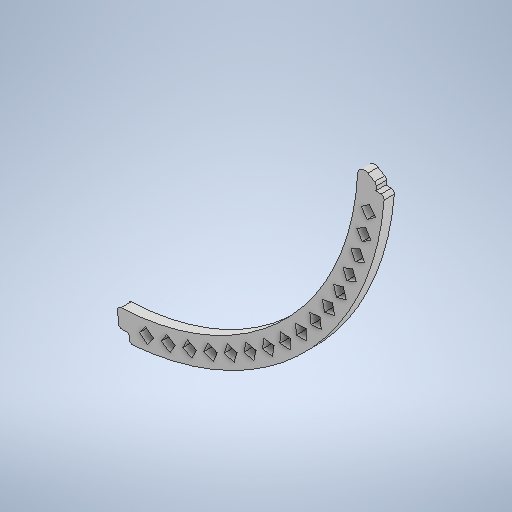
# Autodesk Inventor part: shim_cartridge_V4
Saved by Autodesk Inventor 2025.2 (Build 292293000, 293)
## iProperties
Created: 2024-04-08
Part Number: shim_cartridge_V4
Material: Generic
Document SubType Name: Modeling
Designer: Joshua Harper
Density: 1 g/cm^3
Appearance: Default
Author: Joshua Harper
Autodesk Inventor part; units mm, degrees
ref_plane "YZ Plane" through (0, 0, 0) normal (1, 0, 0) x (0, 1, 0)
ref_plane "XZ Plane" through (0, 0, 0) normal (0, 1, 0) x (-1, 0, 0)
ref_plane "XY Plane" through (0, 0, 0) normal (0, 0, 1) x (1, 0, 0)
sketch "Sketch1" plane through (0, 0, 0) normal (0, 0, 1) x (1, 0, 0)
  arc A0 (5.6926, -80.7997) -> (80.8293, -5.2553) centre (0, 0) ccw
  arc A1 (2.1409, -72.9686) -> (72.998, -0.5377) centre (0, 0) ccw
  line L0 (72.998, -0.5377) -> (80.8095, -0.5953) construction
  line L1 (0, 0) -> (0, 0) construction
  line L2 (2.1409, -72.9686) -> (2.5169, -78.3059)
  line L3 (2.5169, -78.3059) -> (5.5169, -78.3059)
  line L4 (5.5169, -78.3059) -> (5.6926, -80.7997)
  line L5 (78.412, -3.7169) -> (72.998, -0.5377)
  line L6 (78.3059, -5.5169) -> (80.7997, -5.6926)
  arc A2 (78.3059, -5.5169) -> (78.412, -3.7169) centre (0, 0) ccw
  line L7 (0, 0) -> (0, -120.2528) construction
  line L8 (0, 0) -> (5.9355, -84.2471) construction
  line L9 (0, 0) -> (88.2589, 0) construction
  line L10 (0, 0) -> (93.5685, -6.5922) construction
  line L11 (72.998, -0.5377) -> (0, 0) construction
  dimension "d0" = 162
  dimension "d1" = 146
  dimension "d38" = 2.5
  dimension "d39" = 3
  dimension "d40" = 30
  dimension "d52" = 78.5
  dimension "d53" = 1.8
  dimension "d55" = 4.03
  dimension "d57" = 4.03
  constraints: 24 end point, 7 point on circle, 5 coincident, 3 centre point, 3 collinear, 2 horizontal, 2 line through centre, 2 vertical, 1 concentric
  measures "d0" diameter of A0
  measures "d1" diameter of A1
  measures "d38" distance of L4.end L3.end
  measures "d39" distance of L2.end L3.end
  measures "d40" angle of L0 L5
  measures "d52" radius of A2
  measures "d53" vertical distance of L5.start L6.start
  measures "d55" angle of L8 L7
  measures "d57" angle of L9 L10
extrude "Extrusion1" add sketch "Sketch1" along normal blind 3
fillet "Fillet6" radius 2 1 edges at (72.998, -0.5377, 1.5)
sketch "Sketch5" plane through (0, 0, 3) normal (0, 0, 1) x (1, 0, 0)
  line L0 (10.4211, -74.15) -> (12.817, -75.9554)
  line L1 (12.817, -75.9554) -> (11.0116, -78.3513)
  line L2 (11.0116, -78.3513) -> (8.6157, -76.5459)
  line L3 (8.6157, -76.5459) -> (10.4211, -74.15)
  line L4 (0, 0) -> (11.0116, -78.3513) construction
  line L5 (12.817, -75.9554) -> (8.6157, -76.5459) construction
  line L6 (0, 0) -> (0, -125.3413) construction
  line L7 (15.0785, -75.539) -> (16.6742, -72.9985)
  line L8 (16.6742, -72.9985) -> (19.2146, -74.5942)
  line L9 (19.2146, -74.5942) -> (17.619, -77.1347)
  line L10 (17.619, -77.1347) -> (15.0785, -75.539)
  line L11 (21.4327, -73.9874) -> (22.8071, -71.3208)
  line L12 (22.8071, -71.3208) -> (25.4737, -72.6952)
  line L13 (25.4737, -72.6952) -> (24.0993, -75.3618)
  line L14 (24.0993, -75.3618) -> (21.4327, -73.9874)
  line L15 (27.6323, -71.9024) -> (28.7755, -69.1288)
  line L16 (28.7755, -69.1288) -> (31.5492, -70.272)
  line L17 (31.5492, -70.272) -> (30.406, -73.0456)
  line L18 (30.406, -73.0456) -> (27.6323, -71.9024)
  line L19 (33.6327, -69.2989) -> (34.5365, -66.4383)
  line L20 (34.5365, -66.4383) -> (37.3971, -67.3421)
  line L21 (37.3971, -67.3421) -> (36.4933, -70.2027)
  line L22 (36.4933, -70.2027) -> (33.6327, -69.2989)
  line L23 (39.3906, -66.1958) -> (40.0484, -63.2688)
  line L24 (40.0484, -63.2688) -> (42.9754, -63.9266)
  line L25 (42.9754, -63.9266) -> (42.3176, -66.8536)
  line L26 (42.3176, -66.8536) -> (39.3906, -66.1958)
  line L27 (44.8644, -62.6154) -> (45.2716, -59.6431)
  line L28 (45.2716, -59.6431) -> (48.2438, -60.0503)
  line L29 (48.2438, -60.0503) -> (47.8367, -63.0225)
  line L30 (47.8367, -63.0225) -> (44.8644, -62.6154)
  line L31 (50.0148, -58.5834) -> (50.1683, -55.5874)
  line L32 (50.1683, -55.5874) -> (53.1644, -55.7409)
  line L33 (53.1644, -55.7409) -> (53.0109, -58.737)
  line L34 (53.0109, -58.737) -> (50.0148, -58.5834)
  line L35 (54.8046, -54.1291) -> (54.7033, -51.1308)
  line L36 (54.7033, -51.1308) -> (57.7016, -51.0296)
  line L37 (57.7016, -51.0296) -> (57.8028, -54.0279)
  line L38 (57.8028, -54.0279) -> (54.8046, -54.1291)
  line L39 (59.1991, -49.2845) -> (58.8439, -46.3056)
  line L40 (58.8439, -46.3056) -> (61.8228, -45.9504)
  line L41 (61.8228, -45.9504) -> (62.178, -48.9293)
  line L42 (62.178, -48.9293) -> (59.1991, -49.2845)
  line L43 (63.1669, -44.0845) -> (62.5602, -41.1465)
  line L44 (62.5602, -41.1465) -> (65.4982, -40.5399)
  line L45 (65.4982, -40.5399) -> (66.1049, -43.4779)
  line L46 (66.1049, -43.4779) -> (63.1669, -44.0845)
  line L47 (66.6792, -38.5667) -> (65.8254, -35.6907)
  line L48 (65.8254, -35.6907) -> (68.7014, -34.837)
  line L49 (68.7014, -34.837) -> (69.5551, -37.713)
  line L50 (69.5551, -37.713) -> (66.6792, -38.5667)
  line L51 (69.7107, -32.7708) -> (68.616, -29.9776)
  line L52 (68.616, -29.9776) -> (71.4092, -28.883)
  line L53 (71.4092, -28.883) -> (72.5038, -31.6761)
  line L54 (72.5038, -31.6761) -> (69.7107, -32.7708)
  line L55 (72.2395, -26.7386) -> (70.9119, -24.0483)
  line L56 (70.9119, -24.0483) -> (73.6021, -22.7207)
  line L57 (73.6021, -22.7207) -> (74.9298, -25.4109)
  line L58 (74.9298, -25.4109) -> (72.2395, -26.7386)
  line L59 (74.2475, -20.5136) -> (72.6964, -17.9457)
  line L60 (72.6964, -17.9457) -> (75.2643, -16.3946)
  line L61 (75.2643, -16.3946) -> (76.8154, -18.9625)
  line L62 (76.8154, -18.9625) -> (74.2475, -20.5136)
  line L63 (75.7202, -14.1407) -> (73.9568, -11.7136)
  line L64 (73.9568, -11.7136) -> (76.3838, -9.9503)
  line L65 (76.3838, -9.9503) -> (78.1472, -12.3773)
  line L66 (78.1472, -12.3773) -> (75.7202, -14.1407)
  line L67 (73.9568, -11.7136) -> (78.1472, -12.3773) construction
  point P0 (10.7163, -76.2506)
  dimension "d43" = 3
  dimension "d44" = 77
  dimension "d45" = 8
  dimension "d48" = 73
  dimension "d58" = 73
  constraints: 136 end point, 3 perpendicular, 2 parallel, 2 point on line, 1 midpoint, 1 vertical, 121 other
  measures "d43" distance of L2.end L0.start
  measures "d44" distance of point (10.716, -76.251) L4.start
  measures "d45" angle of L4 L6
  measures "d58" angle of L67 L4
extrude "Extrusion5" cut sketch "Sketch5" against normal through all
fillet "Fillet7" radius 1 5 edges at (78.412, -3.7169, 1.5) (80.7997, -5.6926, 1.5) (5.6926, -80.7997, 1.5) (2.1409, -72.9686, 1.5) (2.5169, -78.3059, 1.5)
sketch "Sketch3" plane through (0, 0, 3) normal (0, 0, 1) x (1, 0, 0)
  line L0 (10, -73.0753) -> (2.1409, -73.0753) projected
  circle A0 centre (3.5, -73.0753) radius 1.5
  line L1 (2.1409, -72.9686) -> (2.7074, -81.01) construction
  line L2 (2, -77.0253) -> (11.8753, -77.0253) construction
  ellipse E0 centre (3.5, -81.0253) end of major axis (5, -81.0253) minor radius 0.75
  point P0 (0, 0)
  point P1 (5.6926, -80.7997)
  point P2 (2, -73.0753)
  point P3 (5, -73.0753)
  dimension "d15" = 3
  dimension "d16" = 1.5
  dimension "d20" = 0.75
  dimension "d21" = 1.5
  dimension "d22" = 4
  constraints: 2 centre point, 2 end point, 1 horizontal, 1 vertical alignment, 5 other
  measures "d15" diameter of A0
  measures "d22" distance from line of E0.centre L2
sketch "Sketch4" plane through (0, 0, 3) normal (0, 0, 1) x (1, 0, 0)
  line L0 (80.9861, -1.5) -> (70.9842, -1.5) projected
  line L1 (80.9861, -1.5) -> (78.9861, -1.5)
  line L2 (78.9861, -4) -> (80.9012, -4)
  arc A0 (4.9576, -80.8481) -> (80.9861, -1.5) centre (0, 0) ccw projected
  arc A1 (80.9012, -4) -> (80.9861, -1.5) centre (0, 0) ccw
  line L3 (78.9861, -1.5) -> (78.9861, -4)
  line L4 (74.2542, -1.5) -> (70.9842, -1.5)
  arc A2 (10.8472, -70.1665) -> (70.9842, -1.5) centre (0, 0) ccw projected
  arc A3 (70.8727, -4.25) -> (70.9842, -1.5) centre (0, 0) ccw
  line L5 (70.8727, -4.25) -> (74.2542, -4.25)
  line L6 (74.2542, -4.25) -> (74.2542, -1.5)
  point P0 (10, -70.2922)
  dimension "d25" = 2.5
  dimension "d30" = 2
  dimension "d31" = 2.75
  dimension "d32" = 3.27
  constraints: 12 end point, 6 point on circle, 2 centre point, 2 concentric, 2 horizontal, 2 point on line, 1 collinear, 1 perpendicular, 1 vertical
  measures "d25" distance between parallel lines of L2 L0
  measures "d30" distance of L0.start L1.end
  measures "d31" distance between parallel lines of L0 L5
  measures "d32" distance of L0.end L4.start
equation "\"d16\" = 0.5 * d15"
body "Solid1"
